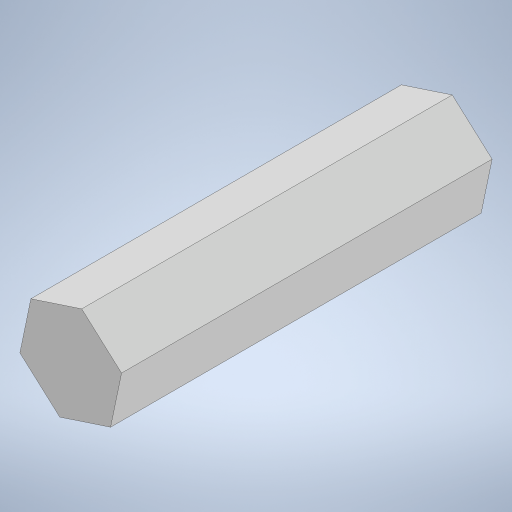
# Autodesk Inventor part: 4-bar intake (2) shaft
Saved by Autodesk Inventor 2023 (Build 270158030, 158C)
## iProperties
Created: 2022-07-19
Part Number: 4-bar intake (2) shaft
Material: Generic
Document SubType Name: Modeling
Designer: rm0990889
Density: 1 g/cm^3
Appearance: Default
Author: rm0990889
Autodesk Inventor part; units mm, degrees
ref_plane "YZ Plane" through (0, 0, 0) normal (1, 0, 0) x (0, 1, 0)
ref_plane "XZ Plane" through (0, 0, 0) normal (0, 1, 0) x (-1, 0, 0)
ref_plane "XY Plane" through (0, 0, 0) normal (0, 0, 1) x (1, 0, 0)
sketch "Sketch1" plane through (0, 0, 0) normal (0, 0, 1) x (1, 0, 0)
  circle A0 centre (0, 0) radius 6.35
  line L0 (6.9674, 2.2843) -> (5.462, -4.8918)
  line L1 (5.462, -4.8918) -> (-1.5054, -7.1761)
  line L2 (-1.5054, -7.1761) -> (-6.9674, -2.2843)
  line L3 (-6.9674, -2.2843) -> (-5.462, 4.8918)
  line L4 (-5.462, 4.8918) -> (1.5054, 7.1761)
  line L5 (1.5054, 7.1761) -> (6.9674, 2.2843)
  point P0 (4.2364, 4.7302)
  dimension "d0" = 12.7
  constraints: 12 end point, 2 coincident, 1 midpoint, 16 other
extrude "Extrusion1" add sketch "Sketch1" along normal blind 50.8
body "Solid1"
